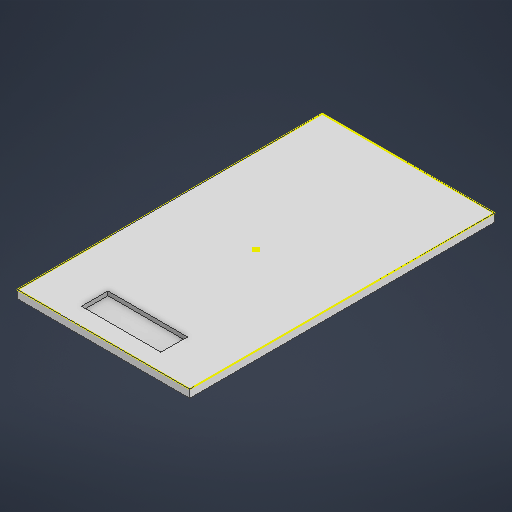
# Autodesk Inventor part: Rear_Port_Slider
Saved by Autodesk Inventor 2026.2 (Build 302298010, 298A)
## iProperties
Created: 2026-05-31
Part Number: Rear_Port_Slider
Material: Generic
Document SubType Name: Modeling
Designer: Srishanth Dhondy
Density: 1 g/cm^3
Appearance: Default
Author: Srishanth Dhondy
Autodesk Inventor part; units mm, degrees
ref_plane "YZ Plane" through (0, 0, 0) normal (1, 0, 0) x (0, 1, 0)
ref_plane "XZ Plane" through (0, 0, 0) normal (0, 1, 0) x (-1, 0, 0)
ref_plane "XY Plane" through (0, 0, 0) normal (0, 0, 1) x (1, 0, 0)
sketch "Sketch1" plane through (0, 0, 0) normal (0, 1, 0) x (-1, 0, 0)
  line L0 (-32.5, -57.5) -> (32.5, -57.5)
  line L1 (32.5, -57.5) -> (32.5, 57.5)
  line L2 (32.5, 57.5) -> (-32.5, 57.5)
  line L3 (-32.5, 57.5) -> (-32.5, -57.5)
  line L4 (-32.5, -57.5) -> (32.5, 57.5) construction
  line L5 (32.5, -57.5) -> (-32.5, 57.5) construction
  point P0 (0, 0)
  dimension "Sliding_Plate_Length" = 65
  dimension "Sliding_Plate_Width" = 115
  constraints: 12 end point, 2 midpoint, 2 parallel, 1 horizontal, 1 perpendicular
  measures "Sliding_Plate_Length" distance of L2.end L1.end
  measures "Sliding_Plate_Width" distance of L1.end L0.end
extrude "Extrusion1" add sketch "Sketch1" along normal blind 3
sketch "Sketch2" plane through (0, 3, 0) normal (0, 1, 0) x (1, 0, 0)
  line L0 (-32.5, 57.5) -> (-32.5, -57.5) projected
  line L1 (-32.5, -57.5) -> (32.5, -57.5) projected
  line L2 (32.5, -57.5) -> (32.5, 57.5) projected
  line L3 (32.5, 57.5) -> (-32.5, 57.5) projected
  point P0 (0, 0)
sketch "Sketch3" plane through (0, 3, 0) normal (0, 1, 0) x (1, 0, 0)
  line L0 (15, -50.862) -> (-15, -50.862)
  line L1 (-15, -50.862) -> (-15, -40.862)
  line L2 (-15, -40.862) -> (15, -40.862)
  line L3 (15, -40.862) -> (15, -50.862)
  line L4 (15, -50.862) -> (-15, -40.862) construction
  line L5 (-15, -50.862) -> (15, -40.862) construction
  point P0 (0, 0)
  point P1 (0, -45.862)
  dimension "d6" = 30
  dimension "d7" = 10
  constraints: 12 end point, 2 midpoint, 2 parallel, 1 horizontal, 1 perpendicular
  measures "d6" distance of L1.end L2.end
  measures "d7" distance of L0.end L1.end
extrude "Extrusion2" cut sketch "Sketch3" against normal blind 1.55
body "Solid1"
